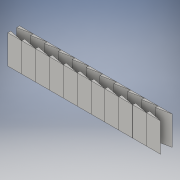
# Autodesk Inventor part: SawTeeth
Saved by Autodesk Inventor 2016 (Build 200138000, 138)
## iProperties
Created: 2016-03-05
Part Number: SawTeeth
Material: Generic
Document SubType Name: Modeling
Designer: yash
Density: 1 g/cm^3
Appearance: Default
Author: yash
Autodesk Inventor part; units mm, degrees
ref_plane "YZ Plane" through (0, 0, 0) normal (1, 0, 0) x (0, 1, 0)
ref_plane "XZ Plane" through (0, 0, 0) normal (0, 1, 0) x (-1, 0, 0)
ref_plane "XY Plane" through (0, 0, 0) normal (0, 0, 1) x (1, 0, 0)
sketch "Sketch3" plane through (0, 0, 0) normal (0, 1, 0) x (-1, 0, 0)
  line L0 (0, 0) -> (1.8764, 0)
  line L1 (1.8764, 0) -> (1.8764, -0.4001)
  line L2 (1.8764, -0.4001) -> (0, 0)
  line L3 (0, 0) -> (0, -0.8001) construction
  line L4 (0, -0.8001) -> (30.0228, -0.8001) construction
  line L5 (0, -1.6002) -> (1.8764, -1.6002)
  line L6 (1.8764, -1.6002) -> (1.8764, -1.2002)
  line L7 (1.8764, -1.2002) -> (0, -1.6002)
  line L8 (5.6356, 0) -> (5.6356, -0.4001)
  line L9 (3.7592, 0) -> (5.6356, 0)
  line L10 (5.6356, -0.4001) -> (3.7592, 0)
  line L11 (5.6356, -1.2002) -> (3.7592, -1.6002)
  line L12 (5.6356, -1.6002) -> (5.6356, -1.2002)
  line L13 (3.7592, -1.6002) -> (5.6356, -1.6002)
  line L14 (9.3948, 0) -> (9.3948, -0.4001)
  line L15 (7.5184, 0) -> (9.3948, 0)
  line L16 (9.3948, -0.4001) -> (7.5184, 0)
  line L17 (9.3948, -1.2002) -> (7.5184, -1.6002)
  line L18 (9.3948, -1.6002) -> (9.3948, -1.2002)
  line L19 (7.5184, -1.6002) -> (9.3948, -1.6002)
  line L20 (13.154, 0) -> (13.154, -0.4001)
  line L21 (11.2776, 0) -> (13.154, 0)
  line L22 (13.154, -0.4001) -> (11.2776, 0)
  line L23 (13.154, -1.2002) -> (11.2776, -1.6002)
  line L24 (13.154, -1.6002) -> (13.154, -1.2002)
  line L25 (11.2776, -1.6002) -> (13.154, -1.6002)
  line L26 (16.9132, 0) -> (16.9132, -0.4001)
  line L27 (15.0368, 0) -> (16.9132, 0)
  line L28 (16.9132, -0.4001) -> (15.0368, 0)
  line L29 (16.9132, -1.2002) -> (15.0368, -1.6002)
  line L30 (16.9132, -1.6002) -> (16.9132, -1.2002)
  line L31 (15.0368, -1.6002) -> (16.9132, -1.6002)
  line L32 (20.6724, 0) -> (20.6724, -0.4001)
  line L33 (18.796, 0) -> (20.6724, 0)
  line L34 (20.6724, -0.4001) -> (18.796, 0)
  line L35 (20.6724, -1.2002) -> (18.796, -1.6002)
  line L36 (20.6724, -1.6002) -> (20.6724, -1.2002)
  line L37 (18.796, -1.6002) -> (20.6724, -1.6002)
  line L38 (1.8796, 0) -> (3.756, 0)
  line L39 (3.756, 0) -> (3.756, -0.4001)
  line L40 (1.8796, -1.6002) -> (3.756, -1.6002)
  line L41 (3.756, -1.2002) -> (1.8796, -1.6002)
  line L42 (3.756, -0.4001) -> (1.8796, 0)
  line L43 (1.8796, 0) -> (1.8796, -0.8001) construction
  line L44 (3.756, -1.6002) -> (3.756, -1.2002)
  line L45 (7.5152, -1.6002) -> (7.5152, -1.2002)
  line L46 (5.6388, -1.6002) -> (7.5152, -1.6002)
  line L47 (7.5152, -1.2002) -> (5.6388, -1.6002)
  line L48 (7.5152, 0) -> (7.5152, -0.4001)
  line L49 (5.6388, 0) -> (7.5152, 0)
  line L50 (7.5152, -0.4001) -> (5.6388, 0)
  line L51 (11.2744, 0) -> (11.2744, -0.4001)
  line L52 (9.398, 0) -> (11.2744, 0)
  line L53 (11.2744, -0.4001) -> (9.398, 0)
  line L54 (9.398, -1.6002) -> (11.2744, -1.6002)
  line L55 (11.2744, -1.6002) -> (11.2744, -1.2002)
  line L56 (11.2744, -1.2002) -> (9.398, -1.6002)
  line L57 (1.8796, -0.8001) -> (31.9024, -0.8001) construction
  line L58 (13.1572, 0) -> (15.0336, 0)
  line L59 (15.0336, -0.4001) -> (13.1572, 0)
  line L60 (13.1572, -1.6002) -> (15.0336, -1.6002)
  line L61 (15.0336, -1.2002) -> (13.1572, -1.6002)
  line L62 (15.0336, -1.6002) -> (15.0336, -1.2002)
  line L63 (15.0336, 0) -> (15.0336, -0.4001)
  line L64 (18.7928, 0) -> (18.7928, -0.4001)
  line L65 (16.9164, 0) -> (18.7928, 0)
  line L66 (18.7928, -0.4001) -> (16.9164, 0)
  line L67 (18.7928, -1.2002) -> (16.9164, -1.6002)
  line L68 (18.7928, -1.6002) -> (18.7928, -1.2002)
  line L69 (16.9164, -1.6002) -> (18.7928, -1.6002)
  dimension "d34" = 1.8764
  dimension "d35" = 0.4001
  dimension "d36" = 0.8001
  dimension "d37" = 30.0228
  dimension "d40" = 3.7592
  dimension "d49" = 1.8796
  constraints: 140 end point, 3 horizontal, 3 symmetric about line, 2 vertical, 1 collinear, 1 perpendicular, 123 other
  measures "d34" distance of L0.start L0.end
  measures "d35" distance of L0.end L1.end
  measures "d36" distance of L0.start L3.end
  measures "d37" distance of L3.end L4.end
  measures "d40" distance of L0.end L8.start
  measures "d49" distance of L0.end L38.end
extrude "Extrusion2" add sketch "Sketch3" along normal blind 3.9116
body "Solid2"
